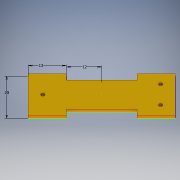
# Autodesk Inventor part: PCB-blank-20x20
Saved by Autodesk Inventor 2017 SP1 (Build 210196100, 196)
## iProperties
Created: 2017-02-03
Part Number: PCB-blank-20x20
Material: Generic
Document SubType Name: Modeling
Designer: Alex
Density: 1 g/cm^3
Appearance: Orange
Author: Alex
Autodesk Inventor part; units mm, degrees
ref_plane "YZ Plane" through (0, 0, 0) normal (1, 0, 0) x (0, 1, 0)
ref_plane "XZ Plane" through (0, 0, 0) normal (0, 1, 0) x (-1, 0, 0)
ref_plane "XY Plane" through (0, 0, 0) normal (0, 0, 1) x (1, 0, 0)
sketch "Sketch1" plane through (0, 0, 0) normal (0, 1, 0) x (-1, 0, 0)
  line L0 (7, 12) -> (10, 12)
  line L1 (-7, 12) -> (-10, 12)
  line L2 (-10, 25) -> (-10, 12)
  line L3 (10, 12) -> (10, 25)
  line L4 (-10, 25) -> (10, 25)
  line L5 (7, 0) -> (-7, 0) construction
  line L6 (-7, 12) -> (-7, 0)
  line L7 (7, 12) -> (7, 0)
  line L8 (-10, 20) -> (0, 20) construction
  line L9 (-10, 20) -> (-5, 20) construction
  line L10 (10, 20) -> (5, 20) construction
  line L11 (7, -12) -> (10, -12)
  line L12 (-7, -12) -> (-10, -12)
  line L13 (-10, -25) -> (-10, -12)
  line L14 (10, -12) -> (10, -25)
  line L15 (-10, -25) -> (10, -25)
  line L16 (-7, -12) -> (-7, 0)
  line L17 (7, -12) -> (7, 0)
  line L18 (-10, -20) -> (0, -20) construction
  line L19 (-10, -20) -> (-5, -20) construction
  line L20 (10, -20) -> (5, -20) construction
  point P0 (0, 0)
  dimension "d39" = 12
  dimension "d40" = 13
  dimension "d41" = 20
  constraints: 42 end point, 11 symmetric about line, 6 point on line, 2 parallel, 1 horizontal, 1 midpoint, 1 perpendicular, 1 vertical
  measures "d39" distance between parallel lines of L0 L5
  measures "d40" distance between parallel lines of L4 L0
  measures "d41" distance between parallel lines of L2 L3
extrude "Extrusion1" add sketch "Sketch1" along normal blind 1
sketch "Sketch2" plane through (0, 1, 0) normal (0, 1, 0) x (1, 0, 0)
  line L0 (-10, -12) -> (-10, -25) projected
  line L1 (-10, -25) -> (-10, -12) projected
  line L2 (-10, -12) -> (-7, -12) projected
  line L3 (7, -12) -> (10, -12) projected
  line L4 (10, -12) -> (10, -25) projected
  line L5 (-7, -12) -> (-7, 12) projected
  line L6 (7, 12) -> (7, -12) projected
  line L7 (10, -25) -> (-10, -25) projected
  line L8 (-7, 12) -> (-10, 12) projected
  line L9 (-10, 12) -> (-10, 25) projected
  line L10 (-10, 25) -> (10, 25) projected
  line L11 (10, 25) -> (10, 12) projected
  line L12 (10, 12) -> (7, 12) projected
  point P0 (0, 0)
  point P1 (-10, -40)
extrude "Extrusion2" add sketch "Sketch2" along normal blind 0.2
hole "Hole3" at (-5, 0, -20) at (5, 0, -20) at (0, 0, 20) direction (0, 1, 0) diameter 1.567 end through all thread size "M2x0.4" class "6H" standard "ISO Metric profile"
body "Solid1"
